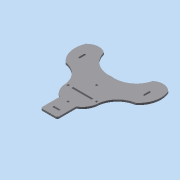
# Autodesk Inventor part: central
Saved by Autodesk Inventor 2015 (Build 190159000, 159)
## iProperties
Created: 2017-10-02
Part Number: central
Material: Generic
Document SubType Name: Modeling
Designer: macbook
Density: 1 g/cm^3
Appearance: Default
Author: macbook
Autodesk Inventor part; units mm, degrees
ref_plane "YZ Plane" through (0, 0, 0) normal (1, 0, 0) x (0, 1, 0)
ref_plane "XZ Plane" through (0, 0, 0) normal (0, 1, 0) x (-1, 0, 0)
ref_plane "XY Plane" through (0, 0, 0) normal (0, 0, 1) x (1, 0, 0)
sketch "Sketch1" plane through (0, 0, 0) normal (0, 0, 1) x (1, 0, 0)
  circle A0 centre (0, 0) radius 50
  arc A1 (-73.4116, 137.5742) -> (0, 87.1574) centre (-8.4976, 153.4397) ccw
  arc A2 (-73.4116, 137.5742) -> (-123.2383, 133.4142) centre (-96.0994, 108.8375) ccw
  arc A3 (-123.2383, 133.4142) -> (-105.1177, 55.113) centre (-61.0095, 106.5679) ccw
  arc A4 (-49.9992, -0.286) -> (-105.1177, 55.113) centre (-114.9857, -9.8243) ccw
  line L0 (-25, 0) -> (25, 0)
  line L1 (25, 0) -> (25, -100)
  line L2 (25, -100) -> (-25, -100)
  line L3 (-25, -100) -> (-25, 0)
  line L4 (0, 63.4714) -> (21.5005, 63.4714) construction
  line L5 (-99.5328, 106.1382) -> (-94.5328, 106.1382)
  line L6 (-94.5328, 106.1382) -> (-94.5328, 86.1382)
  line L7 (-94.5328, 86.1382) -> (-99.5328, 86.1382)
  line L8 (-99.5328, 86.1382) -> (-99.5328, 106.1382)
  arc A5 (0, 87.1574) -> (73.4116, 137.5742) centre (8.4976, 153.4397) ccw
  arc A6 (123.2383, 133.4142) -> (73.4116, 137.5742) centre (96.0994, 108.8375) ccw
  arc A7 (105.1177, 55.113) -> (123.2383, 133.4142) centre (61.0095, 106.5679) ccw
  arc A8 (105.1177, 55.113) -> (49.9992, -0.286) centre (114.9857, -9.8243) ccw
  line L9 (99.5328, 106.1382) -> (94.5328, 106.1382)
  line L10 (94.5328, 106.1382) -> (94.5328, 86.1382)
  line L11 (94.5328, 86.1382) -> (99.5328, 86.1382)
  line L12 (99.5328, 86.1382) -> (99.5328, 106.1382)
  line L13 (49.9992, -0.286) -> (-49.9992, -0.286)
  line L14 (-7.7212, -92.2433) -> (-3.7298, -89.2319)
  line L15 (-3.7298, -89.2319) -> (-15.7757, -73.2664)
  line L16 (-15.7757, -73.2664) -> (-19.7671, -76.2779)
  line L17 (-19.7671, -76.2779) -> (-7.7212, -92.2433)
  line L18 (7.7212, -92.2433) -> (3.7298, -89.2319)
  line L19 (3.7298, -89.2319) -> (15.7757, -73.2664)
  line L20 (15.7757, -73.2664) -> (19.7671, -76.2779)
  line L21 (19.7671, -76.2779) -> (7.7212, -92.2433)
  dimension "d0" = 100
  dimension "d4" = 50
  dimension "d5" = 50
  dimension "d6" = 100
  dimension "d8" = 5
  dimension "d9" = 20
  dimension "d10" = 5
  dimension "d11" = 20
  dimension "d12" = 5
  constraints: 44 end point, 16 point on circle, 8 centre point, 4 horizontal, 4 parallel, 4 perpendicular, 1 coincident, 3 other
  measures "d4" distance of A1.start A2.end
  measures "d5" distance of L1.end L2.end
  measures "d6" distance of L0.end L1.end
  measures "d8" distance of L6.end L7.end
  measures "d9" distance of L5.end L6.end
  measures "d10" distance of L14.start L14.end
  measures "d11" distance of L14.end L15.end
  measures "d12" distance of L15.end L16.end
extrude "Extrusion2" add sketch "Sketch1" along normal blind 5.5 contours A0 L13 L1 L0 L3 | A0 A4 A3 A2 A1 A5 A6 A7 A8 | L13 L3 A0 | A0 L1 L13 | L3 L13 L1 A0 | A0 L1 L2 L3 | L3 L0 L1 L13 | L17 L16 L15 L14 | L18 L19 L20 L21
fillet "Fillet4" radius 2 4 edges at (-99.5328, 106.1382, 2.75) (-94.5328, 106.1382, 2.75) (-94.5328, 86.1382, 2.75) (-99.5328, 86.1382, 2.75)
fillet "Fillet5" radius 2 4 edges at (99.5328, 86.1382, 2.75) (99.5328, 106.1382, 2.75) (94.5328, 106.1382, 2.75) (94.5328, 86.1382, 2.75)
sketch "Sketch2" plane through (0, 0, 5.5) normal (0, 0, 1) x (1, 0, 0)
  line L0 (-10, -80) -> (10, -80)
  line L1 (10, -80) -> (10, -75)
  line L2 (10, -75) -> (-10, -75)
  line L3 (-10, -75) -> (-10, -80)
  point P0 (0, 0)
  dimension "d20" = 20
  dimension "d21" = 5
  constraints: 8 end point, 2 parallel, 1 horizontal, 1 perpendicular
  measures "d20" distance of L2.end L1.end
  measures "d21" distance of L1.end L0.end
extrude "Extrusion3" cut sketch "Sketch2" against normal blind 5.5
fillet "Fillet6" radius 5 2 edges at (25, -100, 2.75) (-25, -100, 2.75)
fillet "Fillet7" radius 2 4 edges at (-10, -75, 2.75) (-10, -80, 2.75) (10, -80, 2.75) (10, -75, 2.75)
fillet "Fillet8" radius 2 2 edges at (-105.1177, 55.113, 2.75) (105.1177, 55.113, 2.75)
sketch "Sketch3" plane through (0, 0, 5.5) normal (0, 0, 1) x (1, 0, 0)
  line L0 (40, 2.7) -> (45, 2.7)
  line L1 (45, 2.7) -> (45, -2.7)
  line L2 (45, -2.7) -> (40, -2.7)
  line L3 (40, -2.7) -> (40, 2.7)
  line L4 (-2.7, 40) -> (-2.7, 45)
  line L5 (-2.7, 45) -> (2.7, 45)
  line L6 (2.7, 45) -> (2.7, 40)
  line L7 (2.7, 40) -> (-2.7, 40)
  line L8 (-40, -2.7) -> (-45, -2.7)
  line L9 (-45, -2.7) -> (-45, 2.7)
  line L10 (-45, 2.7) -> (-40, 2.7)
  line L11 (-40, 2.7) -> (-40, -2.7)
  line L12 (2.7, -40) -> (2.7, -45)
  line L13 (2.7, -45) -> (-2.7, -45)
  line L14 (-2.7, -45) -> (-2.7, -40)
  line L15 (-2.7, -40) -> (2.7, -40)
  point P0 (0, 0)
  point P1 (0, 0)
  dimension "d29" = 5
  dimension "d30" = 5.4
  dimension "d31" = 360
  constraints: 32 end point, 2 parallel, 1 horizontal, 1 perpendicular, 33 other
  measures "d29" distance of L1.end L3.start
  measures "d30" distance of L1.start L1.end
extrude "Extrusion4" cut sketch "Sketch3" against normal blind 5.5
sketch "Sketch4" plane through (0, 0, 5.5) normal (0, 0, 1) x (1, 0, 0)
  line L0 (30, 2.7) -> (-30, 2.7)
  line L1 (-30, 2.7) -> (-30, -2.7)
  line L2 (-30, -2.7) -> (30, -2.7)
  line L3 (30, -2.7) -> (30, 2.7)
  point P0 (0, 0)
  dimension "d34" = 60
  dimension "d35" = 5.4
  constraints: 8 end point, 2 parallel, 1 horizontal, 1 perpendicular
  measures "d34" distance of L2.end L1.end
  measures "d35" distance of L1.end L0.end
extrude "Extrusion5" cut sketch "Sketch4" against normal blind 10
body "Solid2"
